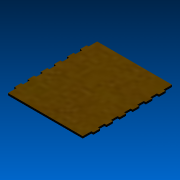
# Autodesk Inventor part: incline
Saved by Autodesk Inventor 2013 SP2 (Build 170200200, 200)
## iProperties
Created: 2015-09-15
Part Number: incline
Material: Generic
Document SubType Name: Modeling
Designer: jeanfrancois
Density: 1 g/cm^3
Author: jeanfrancois
Autodesk Inventor part; units mm, degrees
ref_plane "YZ Plane" through (0, 0, 0) normal (1, 0, 0) x (0, 1, 0)
ref_plane "XZ Plane" through (0, 0, 0) normal (0, 1, 0) x (-1, 0, 0)
ref_plane "XY Plane" through (0, 0, 0) normal (0, 0, 1) x (1, 0, 0)
sketch "Esquisse1" plane through (0, 0, 0) normal (0, 0, 1) x (1, 0, 0)
  line L0 (-63.3507, 41.3748) -> (-66.3507, 41.3748)
  line L1 (-63.3507, 51.3748) -> (-66.3507, 51.3748)
  line L2 (-63.3507, 31.3748) -> (-66.3507, 31.3748)
  line L3 (-63.3507, 21.3748) -> (-66.3507, 21.3748)
  line L4 (-63.3507, 11.3748) -> (-66.3507, 11.3748)
  line L5 (-63.3507, 1.3748) -> (-66.3507, 1.3748)
  line L6 (-63.3507, -8.6252) -> (-66.3507, -8.6252)
  line L7 (-63.3507, -18.6252) -> (-66.3507, -18.6252)
  line L8 (-63.3507, -28.6252) -> (-66.3507, -28.6252)
  line L9 (-63.3507, -38.6252) -> (-66.3507, -38.6252)
  line L10 (53.6493, -48.6252) -> (53.6493, -58.6252)
  line L11 (50.6493, -58.6252) -> (53.6493, -58.6252)
  line L12 (50.6493, -58.6252) -> (50.6493, -71.6252)
  line L13 (50.6493, -48.6252) -> (53.6493, -48.6252)
  line L14 (50.6493, 41.3748) -> (53.6493, 41.3748)
  line L15 (50.6493, 51.3748) -> (53.6493, 51.3748)
  line L16 (50.6493, 64.3748) -> (50.6493, 51.3748)
  line L17 (53.6493, 51.3748) -> (53.6493, 41.3748)
  line L18 (50.6493, -38.6252) -> (50.6493, -48.6252)
  line L19 (50.6493, -38.6252) -> (53.6493, -38.6252)
  line L20 (53.6493, -28.6252) -> (53.6493, -38.6252)
  line L21 (50.6493, -18.6252) -> (50.6493, -28.6252)
  line L22 (50.6493, -28.6252) -> (53.6493, -28.6252)
  line L23 (50.6493, -18.6252) -> (53.6493, -18.6252)
  line L24 (53.6493, -8.6252) -> (53.6493, -18.6252)
  line L25 (50.6493, 1.3748) -> (50.6493, -8.6252)
  line L26 (50.6493, -8.6252) -> (53.6493, -8.6252)
  line L27 (50.6493, 21.3748) -> (50.6493, 11.3748)
  line L28 (50.6493, 1.3748) -> (53.6493, 1.3748)
  line L29 (53.6493, 11.3748) -> (53.6493, 1.3748)
  line L30 (50.6493, 11.3748) -> (53.6493, 11.3748)
  line L31 (50.6493, 31.3748) -> (53.6493, 31.3748)
  line L32 (53.6493, 31.3748) -> (53.6493, 21.3748)
  line L33 (50.6493, 41.3748) -> (50.6493, 31.3748)
  line L34 (50.6493, 21.3748) -> (53.6493, 21.3748)
  line L35 (-63.3507, 64.3748) -> (-63.3507, 51.3748)
  line L36 (50.6493, 64.3748) -> (-63.3507, 64.3748)
  line L37 (50.6493, -71.6252) -> (-63.3507, -71.6252)
  line L38 (-63.3507, 41.3748) -> (-63.3507, 31.3748)
  line L39 (-66.3507, 51.3748) -> (-66.3507, 41.3748)
  line L40 (-66.3507, 31.3748) -> (-66.3507, 21.3748)
  line L41 (-66.3507, 11.3748) -> (-66.3507, 1.3748)
  line L42 (-63.3507, 1.3748) -> (-63.3507, -8.6252)
  line L43 (-66.3507, -8.6252) -> (-66.3507, -18.6252)
  line L44 (-63.3507, -18.6252) -> (-63.3507, -28.6252)
  line L45 (-66.3507, -28.6252) -> (-66.3507, -38.6252)
  line L46 (-63.3507, -38.6252) -> (-63.3507, -48.6252)
  line L47 (-63.3507, -48.6252) -> (-66.3507, -48.6252)
  line L48 (-63.3507, -58.6252) -> (-63.3507, -71.6252)
  line L49 (-63.3507, -58.6252) -> (-66.3507, -58.6252)
  line L50 (-66.3507, -48.6252) -> (-66.3507, -58.6252)
  line L51 (-63.3507, 21.3748) -> (-63.3507, 11.3748)
  point P0 (0, 0)
  constraints: 104 end point
extrude "Extrusion1" add sketch "Esquisse1" along normal blind 3
